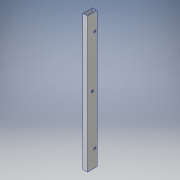
# Autodesk Inventor part: 1x2x28
Saved by Autodesk Inventor 2016 (Build 200138000, 138)
## iProperties
Created: 2016-01-16
Part Number: 1x2x28
Material: Aluminum 6061
Document SubType Name: Modeling
Designer: gus
Density: 2.7 g/cm^3
Appearance: Aluminum - Flat
Mass: 845.202 g
Surface Area: 1988.36 cm^2
Volume: 313.038 cm^3
Author: gus
Autodesk Inventor part; units mm, degrees
ref_plane "YZ Plane" through (0, 0, 0) normal (1, 0, 0) x (0, 1, 0)
ref_plane "XZ Plane" through (0, 0, 0) normal (0, 1, 0) x (-1, 0, 0)
ref_plane "XY Plane" through (0, 0, 0) normal (0, 0, 1) x (1, 0, 0)
sketch "Sketch1" plane through (0, 0, 0) normal (0, 1, 0) x (-1, 0, 0)
  line L0 (0, 0) -> (25.4, 0)
  line L1 (25.4, 0) -> (25.4, -50.8)
  line L2 (25.4, -50.8) -> (0, -50.8)
  line L3 (0, -50.8) -> (0, 0)
  line L4 (3.175, -3.175) -> (22.225, -3.175)
  line L5 (22.225, -3.175) -> (22.225, -47.625)
  line L6 (22.225, -47.625) -> (3.175, -47.625)
  line L7 (3.175, -47.625) -> (3.175, -3.175)
  dimension "d0" = 25.4
  dimension "d1" = 50.8
  dimension "d2" = 3.175
  constraints: 16 end point, 4 parallel, 2 perpendicular, 1 horizontal, 3 other
  measures "d0" distance of L1.end L2.end
  measures "d1" distance of L0.end L1.end
  measures "d2" distance between parallel lines of L3 L7
extrude "Extrusion1" add sketch "Sketch1" along normal blind 711.2
sketch "Sketch2" plane through (-25.4, 0, -50.8) normal (-1, 0, 0) x (0, 0, 1)
  circle A0 centre (25.4, 355.6) radius 6.35
  line L0 (0, 711.2) -> (50.8, 711.2) projected
  line L1 (0, 0) -> (0, 711.2) projected
  circle A1 centre (12.7, 622.3) radius 6.35
  line L2 (50.8, 0) -> (50.8, 711.2) projected
  circle A2 centre (12.7, 88.9) radius 6.35
  line L3 (0, 88.9) -> (50.8, 88.9) construction
  line L4 (50.8, 0) -> (50.8, 711.2) projected
  line L5 (0, 622.3) -> (50.8, 622.3) construction
  dimension "d5" = 12.7
  dimension "d6" = 355.6
  dimension "d7" = 25.4
  dimension "d10" = 12.7
  dimension "d11" = 38.1
  dimension "d13" = 12.7
  dimension "d14" = 38.1
  dimension "d16" = 266.7
  dimension "d17" = 266.7
  constraints: 6 point on line, 4 end point, 3 centre point, 1 horizontal, 1 perpendicular
  measures "d5" diameter of A0
  measures "d6" distance from line of A0.centre L0
  measures "d7" distance from line of L1 A0.centre
  measures "d10" diameter of A1
  measures "d11" distance from line of L2 A1.centre
  measures "d13" diameter of A2
  measures "d14" distance from line of L2 A2.centre
  measures "d16" distance from line of A0.centre L3
  measures "d17" distance from line of A0.centre L5
extrude "Extrusion2" cut sketch "Sketch2" against normal blind 25.4
body "Solid1"
